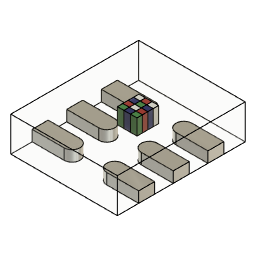
AMS_TCS3472 (Autodesk Fusion 360 design; units mm, degrees)
Autodesk Fusion 360 part; units mm, degrees
sketch "Sketch1" plane through (0, 0, 0) normal (0, 0, 1) x (1, 0, 0) in component "Body"
  line L0 (1, -1.2) -> (-1, -1.2)
  line L1 (-1, -1.2) -> (-1, 1.2)
  line L2 (-1, 1.2) -> (1, 1.2)
  line L3 (1, 1.2) -> (1, -1.2)
  line L4 (1, -1.2) -> (-1, 1.2) construction
  line L5 (-1, -1.2) -> (1, 1.2) construction
  dimension "d1" = 2
  dimension "d2" = 2.4
  constraint horizontal L0
  constraint perpendicular L0 L1
  constraint parallel L0 L2
  constraint parallel L1 L3
  constraint coincident L4 origin
  constraint coincident L5 origin
  measures "d1" distance of L1.end L2.end
  measures "d2" distance of L0.end L1.end
extrude "Extrude1" add sketch "Sketch1" along normal blind 0.65 makes body 1 in component "Body"
sketch "Sketch2" plane through (0, 0, 0.65) normal (0, 0, 1) x (-1, 0, 0) in component "Body"
  line L0 (-1, -1.2) -> (1, -1.2)
  line L1 (1, -1.2) -> (1, 1.2)
  line L2 (1, 1.2) -> (-1, 1.2)
  line L3 (-1, 1.2) -> (-1, -1.2)
  line L4 (0.123, -0.329) -> (-0.246, -0.329)
  line L5 (-0.246, -0.329) -> (-0.246, 0.077)
  line L6 (-0.246, 0.077) -> (0.123, 0.077)
  line L7 (0.123, 0.077) -> (0.123, -0.329)
  dimension "d5" = 0.369
  dimension "d6" = 0.406
  dimension "d7" = 0.877
  dimension "d8" = 0.871
  constraint horizontal L4
  constraint vertical L5
  constraint horizontal L6
  constraint vertical L7
  measures "d5" distance of L4.start L4.end
  measures "d6" distance of L4.end L5.end
  measures "d7" horizontal distance of L0.end L4.start
  measures "d8" vertical distance of L0.end L4.start
extrude "Extrude2" cut sketch "Sketch2" against normal blind 0.295 contours L4 L5 L6 L7 bodies 1 in component "Body"
sketch "Sketch3" plane through (0, 0, 0) normal (0, 0, -1) x (1, 0, 0) in component "Body"
  line L0 (-1, -1.2) -> (1, -1.2)
  line L1 (1, -1.2) -> (1, 1.2)
  line L2 (1, 1.2) -> (-1, 1.2)
  line L3 (-1, 1.2) -> (-1, -1.2)
  line L4 (-1, 0) -> (1, 0) construction
  line L5 (-1, 0.15) -> (-1, -0.15)
  line L6 (-1, 0.15) -> (-0.4, 0.15)
  line L7 (-1, -0.15) -> (-0.4, -0.15)
  line L8 (-0.25, 1.2) -> (-0.25, -1.2) construction
  line L9 (0.25, 1.2) -> (0.25, 1.1)
  line L10 (0.25, 1.1) -> (0.25, -1.2) construction
  line L11 (1, -0.15) -> (1, 0.15)
  line L12 (1, 0.15) -> (0.4, 0.15)
  line L13 (1, -0.15) -> (0.9731, -0.15)
  line L14 (0.9731, -0.15) -> (0.4, -0.15)
  arc A0 (0.4, 0.15) -> (0.4, -0.15) centre (0.4, 0) ccw
  arc A1 (-0.4, -0.15) -> (-0.4, 0.15) centre (-0.4, 0) ccw
  line L15 (-1, 0.65) -> (1, 0.65) construction
  line L16 (-1, -0.65) -> (1, -0.65) construction
  line L17 (1, 0.8) -> (1, 0.5)
  line L18 (1, -0.5) -> (1, -0.8)
  line L19 (-1, 0.8) -> (-1, 0.5)
  line L20 (-1, -0.5) -> (-1, -0.8)
  line L21 (1, 0.8) -> (0.9979, 0.8)
  line L22 (0.9979, 0.8) -> (0.4, 0.8)
  line L23 (1, -0.5) -> (0.4, -0.5)
  line L24 (-1, 0.8) -> (-0.4, 0.8)
  line L25 (-1, 0.5) -> (-0.4, 0.5)
  arc A2 (-0.4, 0.5) -> (-0.4, 0.8) centre (-0.4, 0.65) ccw
  arc A3 (0.4, 0.8) -> (0.401, 0.5) centre (0.4, 0.65) ccw
  arc A4 (0.4, -0.5) -> (0.4, -0.8) centre (0.4, -0.65) ccw
  line L26 (0.4, -0.8) -> (1, -0.8)
  line L27 (-1, -0.5) -> (-0.25, -0.5)
  line L28 (-1, -0.8) -> (-0.25, -0.8)
  line L29 (-0.25, -0.8) -> (-0.25, -0.5)
  line L30 (0.401, 0.5) -> (1, 0.5)
  dimension "d13" = 0.3
  dimension "d16" = 0.75
  dimension "d18" = 0.75
  dimension "d19" = 0.3
  dimension "d20" = 0.15
  dimension "d21" = 0.65
  dimension "d22" = 0.65
  dimension "d23" = 0.6
  dimension "d24" = 0.6
  dimension "d25" = 0.6
  dimension "d26" = 0.6
  constraint midpoint L3 L4.start
  constraint midpoint L1 L4.end
  constraint coincident L3 L5.start
  constraint coincident L3 L5.end
  constraint parallel L3 L5
  constraint symmetric L4 L5.start L5.end
  constraint perpendicular L5 L6
  constraint perpendicular L5 L7
  constraint equal L6 L7
  constraint coincident L2 L8.start
  constraint coincident L0 L8.end
  constraint perpendicular L0 L8
  constraint coincident L2 L9.start
  constraint perpendicular L2 L9
  constraint coincident L0 L10.end
  constraint perpendicular L0 L10
  constraint coincident L1 L11.start
  constraint coincident L1 L11.end
  constraint parallel L1 L11
  constraint symmetric L4 L11.start L11.end
  constraint perpendicular L11 L12
  constraint perpendicular L1 L13
  constraint perpendicular L1 L14
  constraint coincident L4 A0.centre
  constraint tangent L10 A0
  constraint coincident L4 A1.centre
  constraint tangent L8 A1
  constraint coincident L1 L15.end
  constraint perpendicular L1 L15
  constraint coincident L3 L16.start
  constraint coincident L1 L16.end
  constraint perpendicular L3 L16
  constraint coincident L1 L17.start
  constraint coincident L1 L17.end
  constraint parallel L1 L17
  constraint coincident L1 L18.start
  constraint coincident L1 L18.end
  constraint perpendicular L16 L18
  constraint coincident L3 L19.start
  constraint coincident L3 L19.end
  constraint parallel L3 L19
  constraint coincident L3 L20.start
  constraint coincident L3 L20.end
  constraint perpendicular L4 L20
  constraint symmetric L15 L19.start L19.end
  constraint symmetric L15 L17.start L17.end
  constraint symmetric L16 L18.start L18.end
  constraint symmetric L16 L20.start L20.end
  constraint coincident L15.start L19
  constraint equal L17 L19
  constraint equal L17 L18
  constraint equal L18 L20
  constraint equal L5 L20
  constraint perpendicular L17 L21
  constraint perpendicular L17 L22
  constraint perpendicular L18 L23
  constraint perpendicular L3 L24
  constraint perpendicular L19 L25
  constraint equal L24 L25
  constraint coincident L15 A2.centre
  constraint coincident L15 A3.centre
  constraint coincident L16 A4.centre
  constraint tangent L10 A3
  constraint tangent L10 A4
  constraint tangent L8 A2
  constraint perpendicular L18 L26
  constraint equal L23 L26
  constraint coincident L8 L27.end
  constraint perpendicular L8 L27
  constraint coincident L8 L28.end
  constraint perpendicular L8 L28
  measures "d13" distance of L5.start L5.end
  measures "d16" distance of L2.end L8.start
  measures "d18" distance of L1.end L9.start
  measures "d19" distance of L11.start L11.end
  measures "d20" radius of A1
  measures "d21" distance of L4.end L15.end
  measures "d22" distance of L4.end L16.end
  measures "d23" distance of L11.end L12.end
  measures "d24" distance of L17.start L22.end
  measures "d25" distance of L18.start L23.end
  measures "d26" distance of L19.start L24.end
extrude "Extrude3" cut sketch "Sketch3" against normal blind 0.203 contours L3 L20 L27 L28 L29 | L1 L18 L23 A4 L26 | L3 L5 L6 L7 A1 | L1 L11 L12 L13 L14 A0 | L3 L19 L24 L25 A2 | L1 L17 L21 L22 A3 L30 bodies 1 in component "Body"
extrude "Extrude1'" add 6 faces at (-0.6, -0.6, 0.203) (0.6003, -0.7, 0.203) (0.8, 0.05, 0.203) (-0.6, 0.05, 0.203) (-0.5, 0.7, 0.203) (0.8, 0.7, 0.203) along direction (0, 0, -1) up to surface separate body end surface through (0, 0, 0) normal (0, 0, -1) offset 0 on bodies 1 makes body 2 at (-0.5, 0.7, 0.203) makes body 3 at (0.8, 0.05, 0.203) makes body 4 at (-0.6, -0.6, 0.203) makes body 5 at (0.6003, -0.7, 0.203) makes body 6 at (-0.6, 0.05, 0.203) makes body 7 at (0.8, 0.7, 0.203) in component "Pads"
sketch "Sketch1 (2)" plane through (0, 0, 0.355) normal (0, 0, 1) x (-1, 0, 0) in component "Photodiode"
  line L0 (0.123, 0.077) -> (-0.246, 0.077)
  line L1 (-0.246, 0.077) -> (-0.246, -0.329)
  line L2 (-0.246, -0.329) -> (0.123, -0.329)
  line L3 (0.123, -0.329) -> (0.123, 0.077)
  line L4 (0.123, -0.329) -> (0, -0.329)
  line L5 (0, -0.329) -> (0, -0.2275)
  line L6 (0, -0.2275) -> (0.123, -0.2275)
  line L7 (0.123, -0.2275) -> (0.123, -0.329)
  line L8 (-0.246, -0.329) -> (-0.123, -0.329)
  line L9 (-0.123, -0.329) -> (-0.123, -0.2275)
  line L10 (-0.123, -0.2275) -> (-0.246, -0.2275)
  line L11 (-0.246, -0.2275) -> (-0.246, -0.329)
  line L12 (0, -0.126) -> (-0.123, -0.126)
  line L13 (-0.123, -0.126) -> (-0.123, -0.0245)
  line L14 (-0.123, -0.0245) -> (0, -0.0245)
  line L15 (0, -0.0245) -> (0, -0.126)
  dimension "d33" = 0.369
  dimension "d34" = 0.406
  dimension "d35" = 0.123
  dimension "d36" = 0.1015
  dimension "d37" = 0.1015
  constraint horizontal L4
  constraint vertical L5
  constraint horizontal L6
  constraint vertical L7
  constraint coincident L2.end L3.start
  constraint horizontal L8
  constraint vertical L9
  constraint horizontal L10
  constraint vertical L11
  constraint coincident L1.end L2.start
  constraint equal L4 L8
  constraint equal L7 L11
  constraint horizontal L12
  constraint vertical L13
  constraint horizontal L14
  constraint vertical L15
  constraint collinear L9 L13
  constraint collinear L5 L15
  constraint equal L11 L13
  measures "d33" distance of L1.end L2.end
  measures "d34" distance of L0.start L2.end
  measures "d35" distance of L2.end L4.end
  measures "d36" distance of L2.end L6.end
  measures "d37" distance of L5.end L12.start
extrude "Extrude2'" add sketch "Sketch1 (2)" along normal up to surface (0.295 mm away) separate body contours L2 L3 L4 L5 L6 L7 | L1 L2 L8 L9 L10 L11 | L12 L13 L14 L15 makes body 8 at (-0.041, 0.329, 0.4533) makes body 9 at (0.205, 0.329, 0.4533) makes body 10 at (0.041, 0.126, 0.4533) in component "Photodiode"
sketch "Sketch2 (2)" plane through (0, 0, 0.355) normal (0, 0, 1) x (-1, 0, 0) in component "Photodiode"
  line L0 (0.123, 0.077) -> (-0.246, 0.077)
  line L1 (-0.246, 0.077) -> (-0.246, -0.329)
  line L2 (-0.246, -0.329) -> (0.123, -0.329)
  line L3 (0.123, -0.329) -> (0.123, 0.077)
  line L4 (0, -0.329) -> (-0.123, -0.329)
  line L5 (-0.123, -0.329) -> (-0.123, -0.2275)
  line L6 (-0.123, -0.2275) -> (0, -0.2275)
  line L7 (0, -0.2275) -> (0, -0.329)
  line L8 (-0.123, -0.126) -> (-0.246, -0.126)
  line L9 (-0.246, -0.126) -> (-0.246, -0.0245)
  line L10 (-0.246, -0.0245) -> (-0.123, -0.0245)
  line L11 (-0.123, -0.0245) -> (-0.123, -0.126)
  line L12 (0, -0.126) -> (0.123, -0.126)
  line L13 (0.123, -0.126) -> (0.123, -0.0245)
  line L14 (0.123, -0.0245) -> (0, -0.0245)
  line L15 (0, -0.0245) -> (0, -0.126)
  point P0 (0, -0.2275)
  point P1 (-0.123, -0.2275)
  point P2 (0, -0.329)
  point P3 (-0.123, -0.329)
  point P4 (0.123, -0.2275)
  point P5 (-0.246, -0.2275)
  point P6 (-0.123, -0.126)
  point P7 (0, -0.126)
  point P8 (0, -0.0245)
  point P9 (-0.123, -0.0245)
  constraint horizontal L4
  constraint vertical L5
  constraint horizontal L6
  constraint vertical L7
  constraint coincident P1 L5.end
  constraint coincident P2 L4.start
  constraint horizontal L8
  constraint vertical L9
  constraint horizontal L10
  constraint vertical L11
  constraint coincident L1 L9.end
  constraint coincident P6 L8.start
  constraint coincident P9 L10.end
  constraint horizontal L12
  constraint vertical L13
  constraint horizontal L14
  constraint vertical L15
  constraint coincident L3 L13.end
  constraint coincident P7 L12.start
  constraint coincident P8 L14.end
extrude "Extrude4" add sketch "Sketch2 (2)" along normal up to surface (0.295 mm away) separate body contours L3 L12 L13 L14 L15 | L1 L8 L9 L10 L11 | L2 L4 L5 L6 L7 makes body 11 at (0.082, 0.329, 0.4533) makes body 12 at (-0.041, 0.126, 0.4533) makes body 13 at (0.205, 0.0245, 0.4533) in component "Photodiode"
sketch "Sketch3 (2)" plane through (0, 0, 0.355) normal (0, 0, 1) x (-1, 0, 0) in component "Photodiode"
  line L0 (0.123, 0.077) -> (-0.246, 0.077)
  line L1 (-0.246, 0.077) -> (-0.246, -0.329)
  line L2 (-0.246, -0.329) -> (0.123, -0.329)
  line L3 (0.123, -0.329) -> (0.123, 0.077)
  line L4 (0, -0.2275) -> (-0.123, -0.2275)
  line L5 (-0.123, -0.2275) -> (-0.123, -0.126)
  line L6 (-0.123, -0.126) -> (0, -0.126)
  line L7 (0, -0.126) -> (0, -0.2275)
  line L8 (-0.123, -0.0245) -> (-0.246, -0.0245)
  line L9 (-0.246, -0.0245) -> (-0.246, 0.077)
  line L10 (-0.246, 0.077) -> (-0.123, 0.077)
  line L11 (-0.123, 0.077) -> (-0.123, -0.0245)
  line L12 (0, -0.0245) -> (0.123, -0.0245)
  line L13 (0.123, -0.0245) -> (0.123, 0.077)
  line L14 (0.123, 0.077) -> (0, 0.077)
  line L15 (0, 0.077) -> (0, -0.0245)
  point P0 (0, -0.2275)
  point P1 (-0.123, -0.2275)
  point P2 (0, -0.126)
  point P3 (-0.123, -0.126)
  point P4 (0, -0.0245)
  point P5 (0.123, -0.0245)
  point P6 (-0.123, -0.0245)
  point P7 (-0.246, -0.0245)
  constraint horizontal L4
  constraint vertical L5
  constraint horizontal L6
  constraint vertical L7
  constraint coincident P3 L5.end
  constraint coincident P0 L4.start
  constraint horizontal L8
  constraint vertical L9
  constraint horizontal L10
  constraint vertical L11
  constraint coincident L0.end L1.start
  constraint coincident P6 L8.start
  constraint horizontal L12
  constraint vertical L13
  constraint horizontal L14
  constraint vertical L15
  constraint coincident L0.start L3.end
  constraint coincident P4 L12.start
extrude "Extrude5" add sketch "Sketch3 (2)" along normal up to surface (0.295 mm away) separate body contours L0 L3 L12 L13 L14 L15 | L0 L1 L8 L9 L10 L11 | L4 L5 L6 L7 makes body 14 at (0.041, 0.2275, 0.4533) makes body 15 at (-0.041, 0.0245, 0.4533) makes body 16 at (0.164, 0.0245, 0.4533) in component "Photodiode"
sketch "Sketch4" plane through (0, 0, 0.355) normal (0, 0, 1) x (-1, 0, 0) in component "Photodiode"
  line L0 (0.123, 0.077) -> (-0.246, 0.077)
  line L1 (-0.246, 0.077) -> (-0.246, -0.329)
  line L2 (-0.246, -0.329) -> (0.123, -0.329)
  line L3 (0.123, -0.329) -> (0.123, 0.077)
  line L4 (0.123, -0.2275) -> (0, -0.2275)
  line L5 (0, -0.2275) -> (0, -0.126)
  line L6 (0, -0.126) -> (0.123, -0.126)
  line L7 (0.123, -0.126) -> (0.123, -0.2275)
  line L8 (-0.123, -0.2275) -> (-0.246, -0.2275)
  line L9 (-0.246, -0.2275) -> (-0.246, -0.126)
  line L10 (-0.246, -0.126) -> (-0.123, -0.126)
  line L11 (-0.123, -0.126) -> (-0.123, -0.2275)
  line L12 (0, -0.0245) -> (-0.123, -0.0245)
  line L13 (-0.123, -0.0245) -> (-0.123, 0.077)
  line L14 (-0.123, 0.077) -> (0, 0.077)
  line L15 (0, 0.077) -> (0, -0.0245)
  point P0 (0, -0.2275)
  point P1 (0.123, -0.2275)
  point P2 (0.123, -0.126)
  point P3 (0, -0.126)
  point P4 (-0.123, -0.2275)
  point P5 (-0.246, -0.2275)
  point P6 (-0.123, -0.126)
  point P7 (-0.246, -0.126)
  point P8 (0, -0.0245)
  point P9 (0, 0.077)
  point P10 (-0.123, -0.0245)
  point P11 (-0.123, 0.077)
  constraint horizontal L4
  constraint vertical L5
  constraint horizontal L6
  constraint vertical L7
  constraint coincident P3 L5.end
  constraint coincident P1 L4.start
  constraint horizontal L8
  constraint vertical L9
  constraint horizontal L10
  constraint vertical L11
  constraint coincident P7 L9.end
  constraint coincident P4 L8.start
  constraint horizontal L12
  constraint vertical L13
  constraint horizontal L14
  constraint vertical L15
  constraint coincident P11 L13.end
  constraint coincident P8 L12.start
extrude "Extrude6" add sketch "Sketch4" along normal up to surface (0.295 mm away) separate body contours L0 L12 L13 L14 L15 | L3 L4 L5 L6 L7 | L1 L8 L9 L10 L11 makes body 17 at (-0.082, 0.2275, 0.4533) makes body 18 at (0.205, 0.126, 0.4533) makes body 19 at (0.041, 0.0245, 0.4533) in component "Photodiode"
copy_body "CutPasteBodies1" bodies 10 9 8 removing the originals makes body 20 makes body 21 makes body 22 in component "Photodiode_Clear"
copy_body "CutPasteBodies1'" bodies 11 12 13 removing the originals makes body 23 makes body 24 makes body 25 in component "Photodiode_Red"
copy_body "CutPasteBodies1''" bodies 14 15 16 removing the originals makes body 26 makes body 27 makes body 28 in component "Photodiode_Green"
copy_body "CutPasteBodies1'''" bodies 17 19 18 removing the originals makes body 29 makes body 30 makes body 31 in component "Photodiode_Blue"
component "Body" placed x (1, 0, 0) y (0, 1, 0) z (0, 0, 1) at (0, 0, 0)
component "Photodiode" placed x (1, 0, 0) y (0, 1, 0) z (0, 0, 1) at (0, 0, 0)
component "Pads" placed x (1, 0, 0) y (0, 1, 0) z (0, 0, 1) at (0, 0, 0)
component "Photodiode_Clear" placed x (1, 0, 0) y (0, 1, 0) z (0, 0, 1) at (0, 0, 0)
component "Photodiode_Blue" placed x (1, 0, 0) y (0, 1, 0) z (0, 0, 1) at (0, 0, 0)
component "Photodiode_Red" placed x (1, 0, 0) y (0, 1, 0) z (0, 0, 1) at (0, 0, 0)
component "Photodiode_Green" placed x (1, 0, 0) y (0, 1, 0) z (0, 0, 1) at (0, 0, 0)
equation "d18 = d16"
equation "d19 = d13"
equation "d22 = d21"
equation "d24 = d23"
equation "d25 = d23"
equation "d26 = d23"
equation "d35 = 0.369 mm / 3"
equation "d36 = 0.406 mm / 4"
equation "d37 = d36"
